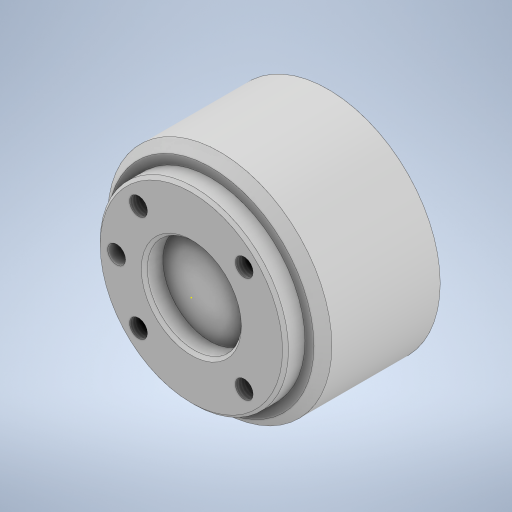
# Autodesk Inventor part: tool-output-flange
Saved by Autodesk Inventor 2024 (Build 280153000, 153)
## iProperties
Created: 2024-09-21
Part Number: tool-output-flange
Material: 一般
Document SubType Name: Modeling
Designer: 1412z
Density: 1 g/cm^3
Appearance: 既定
Author: 1412z
Autodesk Inventor part; units mm, degrees
ref_plane "YZ Plane" through (0, 0, 0) normal (1, 0, 0) x (0, 1, 0)
ref_plane "XZ Plane" through (0, 0, 0) normal (0, 1, 0) x (-1, 0, 0)
ref_plane "XY Plane" through (0, 0, 0) normal (0, 0, 1) x (1, 0, 0)
sketch "スケッチ1" plane through (0, 0, 0) normal (0, 0, 1) x (1, 0, 0)
  circle A0 centre (0, 0) radius 37.5
  dimension "d0" = 75
  constraints: 1 centre point, 1 coincident
  measures "d0" diameter of A0
extrude "押し出し1" add sketch "スケッチ1" along normal blind 45.75
sketch "スケッチ2" plane through (0, 0, 45.75) normal (0, 0, 1) x (1, 0, 0)
  circle A0 centre (0, 0) radius 37.5
  circle A1 centre (0, 0) radius 31.5
  dimension "d3" = 63
  constraints: 2 centre point, 2 coincident
  measures "d3" diameter of A1
extrude "押し出し2" cut sketch "スケッチ2" against normal blind 6.5
chamfer "面取り1" distance 3 angle 45 1 edges at (-37.5, 0, 39.25)
chamfer "面取り2" distance 1 angle 45 1 edges at (-31.5, 0, 45.75)
sketch "スケッチ3" plane through (0, 0, 45.75) normal (0, 0, 1) x (1, 0, 0)
  circle A0 centre (0, 0) radius 15.75
  dimension "d12" = 31.5
  constraints: 1 centre point, 1 coincident
  measures "d12" diameter of A0
extrude "押し出し3" cut sketch "スケッチ3" against normal blind 6.2
chamfer "面取り3" distance 1 angle 45 1 edges at (-15.75, 0, 45.75)
sketch "スケッチ4" plane through (0, 0, 45.75) normal (0, 0, 1) x (1, 0, 0)
  circle A0 centre (-25, 0) radius 3
  point P0 (0, 0)
  dimension "d18" = 6
  constraints: 1 centre point
  measures "d18" diameter of A0
extrude "押し出し4" cut sketch "スケッチ4" against normal blind 6.2
sketch "スケッチ5" plane through (0, 0, 45.75) normal (0, 0, 1) x (1, 0, 0)
  point P0 (0, 0)
sketch "スケッチ6" plane through (0, 0, 45.75) normal (0, 0, 1) x (1, 0, 0)
  circle A0 centre (0, 0) radius 25
  circle A1 centre (0, 0) radius 37.5 projected
  line L0 (0, 0) -> (-17.6777, 17.6777)
  line L1 (0, 0) -> (25, 0) construction
  circle A2 centre (-17.6777, 17.6777) radius 3
  circle A3 centre (17.6777, 17.6777) radius 3
  circle A4 centre (17.6777, -17.6777) radius 3
  circle A5 centre (-17.6777, -17.6777) radius 3
  dimension "d21" = 50
  dimension "d22" = 135
  dimension "d23" = 6
  dimension "d24" = 6
  dimension "d25" = 6
  dimension "d26" = 6
  constraints: 5 centre point, 4 end point, 4 point on circle, 2 coincident, 1 equal length, 1 horizontal
  measures "d21" diameter of A0
  measures "d22" angle of L1 L0
  measures "d23" diameter of A2
  measures "d24" diameter of A3
  measures "d25" diameter of A4
  measures "d26" diameter of A5
extrude "押し出し5" cut sketch "スケッチ6" against normal blind 8 contours A3 A0 | A0 A3 | A4 A0 | A0 A4 | A2 L0 A0 | A0 A2 | A5 A0 | A0 A5 | L0 A2 A0
thread "ねじ1" size "M6x1" class "6H" standard "ANSI Metric M Profile" full length
thread "ねじ2" size "M6x1" class "6H" standard "ANSI Metric M Profile" full length
thread "ねじ3" size "M6x1" class "6H" standard "ANSI Metric M Profile" full length
thread "ねじ4" size "M6x1" class "6H" standard "ANSI Metric M Profile" full length
sketch "スケッチ7" plane through (0, 0, 0) normal (1, 0, 0) x (0, 1, 0)
  circle A0 centre (0, 14.2) radius 4
  point P0 (0, 0)
  dimension "d37" = 8
  constraints: 1 centre point
  measures "d37" diameter of A0
extrude "押し出し6" add sketch "スケッチ7" against normal blind 40
